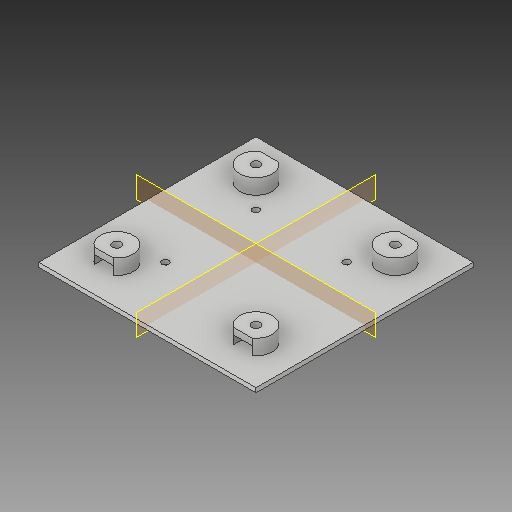
# Autodesk Inventor part: support-balise
Saved by Autodesk Inventor 2019 (Build 230136000, 136)
## iProperties
Created: 2018-04-02
Part Number: support-balise
Material: Générique
Document SubType Name: Modeling
Designer: franc
Density: 1 g/cm^3
Appearance: Par défaut
Author: franc
Autodesk Inventor part; units mm, degrees
ref_plane "YZ Plane" through (0, 0, 0) normal (1, 0, 0) x (0, 1, 0)
ref_plane "XZ Plane" through (0, 0, 0) normal (0, 1, 0) x (-1, 0, 0)
ref_plane "XY Plane" through (0, 0, 0) normal (0, 0, 1) x (1, 0, 0)
sketch "Esquisse1" plane through (0, 0, 0) normal (0, 1, 0) x (-1, 0, 0)
  line L0 (50, 50) -> (-50, 50)
  line L1 (-50, 50) -> (-50, -50)
  line L2 (-50, -50) -> (50, -50)
  line L3 (50, -50) -> (50, 50)
  point P0 (0, 0)
  dimension "d0" = 100
  dimension "d1" = 100
  dimension "d17" = 50
  dimension "d18" = 50
  constraints: 8 end point, 2 parallel, 1 horizontal, 1 perpendicular
  measures "d0" distance of L2.end L0.start
  measures "d1" distance of L1.end L2.end
  measures "d17" distance from line of L1 point (0, 0)
  measures "d18" distance from line of L0 point (0, 0)
extrude "Extrusion1" add sketch "Esquisse1" along normal blind 2
sketch "Esquisse2" plane through (0, 2, 0) normal (0, 1, 0) x (1, 0, 0)
  line L0 (50, -50) -> (50, 50) projected
  line L1 (-50, -50) -> (50, -50) projected
  arc A0 (36.32, -38.1309) -> (27.6597, -38.1165) centre (32, -32) ccw
  line L2 (27.68, -29.4825) -> (32.0203, -27)
  line L3 (32.0203, -27) -> (36.3403, -29.5175)
  line L4 (36.3403, -29.5175) -> (36.32, -34.5175)
  line L5 (27.6597, -34.4825) -> (27.68, -29.4825)
  line L6 (27.6597, -34.4825) -> (27.6597, -38.1165)
  line L7 (36.32, -34.5175) -> (36.32, -38.1309)
  line L8 (53.6963, 0) -> (-74.6388, 0)
  line L9 (0, -61.7794) -> (0, 59.6738)
  arc A1 (-27.6597, -38.1165) -> (-36.32, -38.1309) centre (-32, -32) ccw
  line L10 (-27.68, -29.4825) -> (-32.0203, -27)
  line L11 (-32.0203, -27) -> (-36.3403, -29.5175)
  line L12 (-36.3403, -29.5175) -> (-36.32, -34.5175)
  line L13 (-27.6597, -34.4825) -> (-27.68, -29.4825)
  line L14 (-27.6597, -34.4825) -> (-27.6597, -38.1165)
  line L15 (-36.32, -34.5175) -> (-36.32, -38.1309)
  arc A2 (27.6597, 38.1165) -> (36.32, 38.1309) centre (32, 32) ccw
  line L16 (27.68, 29.4825) -> (32.0203, 27)
  line L17 (32.0203, 27) -> (36.3403, 29.5175)
  line L18 (36.3403, 29.5175) -> (36.32, 34.5175)
  line L19 (27.6597, 34.4825) -> (27.68, 29.4825)
  line L20 (27.6597, 34.4825) -> (27.6597, 38.1165)
  line L21 (36.32, 34.5175) -> (36.32, 38.1309)
  arc A3 (-36.32, 38.1309) -> (-27.6597, 38.1165) centre (-32, 32) ccw
  line L22 (-27.68, 29.4825) -> (-32.0203, 27)
  line L23 (-32.0203, 27) -> (-36.3403, 29.5175)
  line L24 (-36.3403, 29.5175) -> (-36.32, 34.5175)
  line L25 (-27.6597, 34.4825) -> (-27.68, 29.4825)
  line L26 (-27.6597, 34.4825) -> (-27.6597, 38.1165)
  line L27 (-36.32, 34.5175) -> (-36.32, 38.1309)
  point P0 (0, 0)
  dimension "d6" = 18
  dimension "d7" = 18
  dimension "d8" = 15
  dimension "d9" = 5
  constraints: 52 end point, 27 symmetric about line, 8 point on circle, 4 centre point, 4 coincident, 2 vertical, 1 horizontal, 11 other
  measures "d6" distance from line of L1 A0.centre
  measures "d7" distance from line of L0 A0.centre
  measures "d8" diameter of A0
  measures "d9" vertical distance of L5.start L2.start
extrude "Extrusion2" add sketch "Esquisse2" along normal blind 4 contours L7 L4 L3 L2 L5 L6 A0 | L14 L13 L10 L11 L12 L15 A1 | L20 L19 L16 L17 L18 L21 A2 | L27 L24 L23 L22 L25 L26 A3
sketch "Esquisse4" plane through (0, 6, 0) normal (0, 1, 0) x (1, 0, 0)
  arc A0 (36.32, -38.1309) -> (27.6597, -38.1165) centre (32, -32) ccw projected
  line L0 (27.6597, -38.1165) -> (36.3403, -38.1165)
  line L1 (53.7761, 0) -> (-84.9694, 0)
  line L2 (0, -51.9111) -> (0, 71.3221)
  arc A1 (-27.6597, -38.1165) -> (-36.32, -38.1309) centre (-32, -32) ccw
  line L3 (-27.6597, -38.1165) -> (-36.3403, -38.1165)
  arc A2 (27.6597, 38.1165) -> (36.32, 38.1309) centre (32, 32) ccw
  line L4 (27.6597, 38.1165) -> (36.3403, 38.1165)
  arc A3 (-36.32, 38.1309) -> (-27.6597, 38.1165) centre (-32, 32) ccw
  line L5 (-27.6597, 38.1165) -> (-36.3403, 38.1165)
  point P0 (0, 0)
  constraints: 12 end point, 12 symmetric about line, 10 point on circle, 3 centre point, 2 horizontal, 1 vertical, 3 other
extrude "Extrusion3" add sketch "Esquisse4" along normal blind 3
sketch "Esquisse5" plane through (0, 9, 0) normal (0, 1, 0) x (1, 0, 0)
  circle A0 centre (32, -32) radius 2
  arc A1 (36.3403, -38.1165) -> (27.6597, -38.1165) centre (32, -32) ccw projected
  line L0 (0, -51.4977) -> (0, 66.0278)
  line L1 (54.9768, 0) -> (-89.9714, 0)
  circle A2 centre (-32, -32) radius 2
  arc A3 (-27.6597, -38.1165) -> (-36.3403, -38.1165) centre (-32, -32) ccw
  circle A4 centre (32, 32) radius 2
  arc A5 (27.6597, 38.1165) -> (36.3403, 38.1165) centre (32, 32) ccw
  circle A6 centre (-32, 32) radius 2
  arc A7 (-36.3403, 38.1165) -> (-27.6597, 38.1165) centre (-32, 32) ccw
  point P0 (0, 0)
  dimension "d14" = 4
  constraints: 12 symmetric about line, 7 centre point, 6 point on circle, 4 end point, 1 concentric, 1 horizontal, 1 vertical, 6 other
  measures "d14" diameter of A0
extrude "Extrusion4" cut sketch "Esquisse5" against normal through all
ref_plane "Plan de construction3" through (0, 0, 50) normal (1, 0, 0) x (0, 0, -1)
ref_plane "Plan de construction4" through (-50, 0, 0) normal (0, 0, 1) x (1, 0, 0)
sketch "Esquisse6" plane through (0, 0, 0) normal (0, -1, 0) x (1, 0, 0)
  circle A0 centre (20.8597, 20.8597) radius 1.6 projected
  circle A1 centre (20.8597, -20.8597) radius 1.6 projected
  circle A2 centre (-20.8597, 20.8597) radius 1.6 projected
  circle A3 centre (-20.8597, -20.8597) radius 1.6 projected
  point P0 (0, 0)
extrude "Extrusion5" cut sketch "Esquisse6" against normal through all
